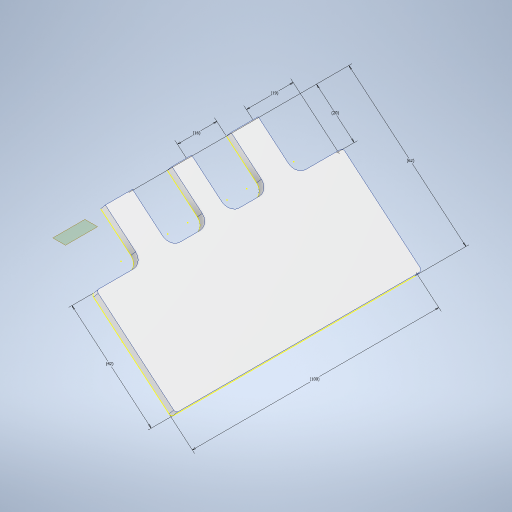
# Autodesk Inventor part: mirror
Saved by Autodesk Inventor 2023.5 (Build 275446000, 446)
## iProperties
Created: 2022-12-26
Part Number: mirror
Material: Aluminium 6061
Document SubType Name: Modeling
Designer: Kamil
Density: 2.7 g/cm^3
Appearance: Aluminium — płaski
Mass: 39.0399 g
Surface Area: 108.154 cm^2
Volume: 14.4592 cm^3
Author: Kamil
Autodesk Inventor part; units mm, degrees
ref_plane "YZ Plane" through (0, 0, 0) normal (1, 0, 0) x (0, 1, 0)
ref_plane "XZ Plane" through (0, 0, 0) normal (0, 1, 0) x (-1, 0, 0)
sketch "Sketch1" plane through (0, 0, 0) normal (0, 0, 1) x (1, 0, 0)
  line L0 (-44.6274, 16.55) -> (3.1619, -23.55) projected
  line L1 (44.6274, -23.55) -> (3.1619, -23.55) projected
  line L2 (44.6274, -23.55) -> (44.6274, -12.55) projected
  line L3 (44.6274, -12.55) -> (28.5274, -12.55) projected
  arc A0 (10.4274, 5.55) -> (28.5274, -12.55) centre (28.5274, 5.55) ccw projected
  line L4 (10.4274, 5.55) -> (10.4274, 16.55) projected
  line L5 (10.4274, 16.55) -> (-44.6274, 16.55) projected
  line L6 (-55.3726, 21.65) -> (-32.3912, 2.3664) projected
  line L7 (-32.3912, 2.3664) -> (-30.4629, 4.6645) projected
  line L8 (-30.4629, 4.6645) -> (-50.7054, 21.65) projected
  line L9 (-50.7054, 21.65) -> (-55.3726, 21.65) projected
  line L10 (-32.3912, 2.3664) -> (12.526, -35.3237)
  line L11 (3.1619, -23.55) -> (14.4544, -33.0256)
  line L12 (14.4544, -33.0256) -> (12.526, -35.3237)
  point P0 (0, 0)
  constraints: 6 end point, 1 perpendicular
ref_plane "Work Plane1" through (-44.6274, -23.55, -100) normal (0, 0, -1) x (0, 1, 0)
extrude "Extrusion1" add sketch "Sketch1" against normal up to surface (100 mm away) contours L0 L11 L12 L10 L7
sketch "Sketch2" plane through (14.4544, -33.0256, -100) normal (0, 0, -1) x (-0.7660444, 0.6427876, 0)
  line L0 (-13.6181, 16.6167) -> (-12.086, 15.3311)
  line L1 (-12.086, 15.3311) -> (12.4819, -5.2838)
  line L2 (0, 0) -> (58.6353, 0) projected
  line L3 (0, -3) -> (0, 0) projected
  line L4 (58.6353, -3) -> (0, -3) projected
  line L5 (58.6353, 0) -> (58.6353, -3) projected
  point P0 (32.3011, 16.0079)
  point P1 (9.7601, -3)
  point P2 (6.1849, 0)
  constraints: 4 end point, 3 other
extrude "Extrusion2" cut sketch "Sketch2" against normal through all contours L1 L4 L3 L2
ref_plane "Work Plane2" through (-55.2717, 8.4367, -43.1782) normal (0, -1, 0) x (1, 0, 0)
sketch "Sketch4" plane through (-32.3912, 2.3664, -100) normal (-0.6427876, -0.7660444, 0) x (0.7660444, -0.6427876, 0)
  line L0 (48.8752, 0) -> (48.8752, 100) projected
  line L1 (0, 100) -> (48.8752, 100) projected
  line L2 (0, 100) -> (0, 0) projected
  line L3 (0, 0) -> (48.8752, 0) projected
  line L4 (-5.8685, 94) -> (-21.784, 94)
  line L5 (43.894, 94) -> (0.9766, 94)
  line L6 (48.8752, 0) -> (48.8752, 100) projected
  line L7 (48.8752, 50) -> (0, 50)
  line L8 (0, 100) -> (0, 0) projected
  line L9 (26.3342, 100) -> (26.3342, 94)
  line L10 (26.3342, 97) -> (26.3342, 96.5)
  circle A0 centre (26.3342, 96.5) radius 1.5
  circle A1 centre (26.3342, 3.5) radius 1.5
  dimension "d6" = 0.5
  dimension "d7" = 3
  constraints: 10 end point, 3 midpoint, 2 centre point, 2 horizontal, 2 point on line, 1 coincident, 1 perpendicular, 1 symmetric about line, 5 other
  measures "d6" distance of L10.start L10.end
  measures "d7" diameter of A0
extrude "Extrusion3" cut sketch "Sketch4" against normal blind 10 contours L9 A0 | L9 A0 | A1
chamfer "Chamfer1" distance 1 angle 45 2 edges at (-13.3671, -13.5967, -3.5) (-13.3671, -13.5967, -96.5)
sketch "Szkic5" plane through (-32.3912, 2.3664, -100) normal (-0.7660444, 0.6427876, 0) x (0, 0, 1)
  line L0 (0, 3) -> (0, 0) projected
  line L1 (100, 0) -> (0, 0) projected
  line L2 (100, 3) -> (100, 0) projected
  line L3 (100, 3) -> (0, 3) projected
  point P0 (100, 19.0079)
extrude "Wyciągnięcie proste4" add sketch "Szkic5" along normal blind 10
sketch "Szkic6" plane through (5.0493, -29.05, -100) normal (-0.6427876, -0.7660444, 0) x (0.7660444, -0.6427876, 0)
  line L0 (-58.8752, 0) -> (-58.8752, 100) projected
  line L1 (-58.8752, 100) -> (0, 100) projected
  line L2 (0, 0) -> (-58.8752, 0) projected
  line L3 (-38.8752, 100) -> (-38.8752, 0)
  line L4 (-38.8752, 50) -> (-58.8752, 50)
  line L5 (-58.8752, 100) -> (-58.8752, 0) projected
  line L6 (-38.8752, 46) -> (-58.8752, 46)
  line L7 (-38.8752, 54) -> (-58.8752, 54)
  line L8 (-38.8752, 81) -> (-58.8752, 81)
  line L9 (-38.8752, 19) -> (-58.8752, 19)
  line L10 (-38.8752, 70) -> (-58.8752, 70)
  line L11 (-38.8752, 30) -> (-58.8752, 30)
  point P0 (-22.541, 100)
  point P1 (-58.8752, 19)
  point P2 (-58.8752, 30)
  point P3 (-58.8752, 46)
  point P4 (-58.8752, 54)
  point P5 (-58.8752, 81)
  dimension "d15" = 20
  dimension "d16" = 4
  dimension "d17" = 4
  dimension "d18" = 19
  dimension "d19" = 19
  dimension "d20" = 11
  dimension "d21" = 11
  constraints: 16 end point, 10 point on line, 5 perpendicular, 2 midpoint, 2 parallel
  measures "d15" distance between parallel lines of L0 L3
  measures "d16" distance between parallel lines of L4 L6
  measures "d17" distance between parallel lines of L4 L7
  measures "d18" distance between parallel lines of L8 L1
  measures "d19" distance between parallel lines of L2 L9
  measures "d20" distance between parallel lines of L9 L11
  measures "d21" distance between parallel lines of L8 L10
extrude "Wyciągnięcie proste5" cut sketch "Szkic6" against normal through all contours L0 L9 L3 L2 | L0 L6 L3 L11 | L0 L10 L3 L7 | L0 L1 L3 L8
fillet "Zaokrąglenie1" radius 4 6 edges at (-23.7666, -2.9124, -19) (-23.7666, -2.9124, -46) (-23.7666, -2.9124, -30) (-23.7666, -2.9124, -54) (-23.7666, -2.9124, -70) (-23.7666, -2.9124, -81)
sketch "Szkic7" plane through (5.0493, -29.05, -100) normal (-0.6427876, -0.7660444, 0) x (0.7660444, -0.6427876, 0)
  circle A0 centre (-22.541, 96.5) radius 2.5 projected
  circle A1 centre (-22.541, 3.5) radius 2.5 projected
  point P0 (-22.541, 100)
extrude "Wyciągnięcie proste6" add sketch "Szkic7" against normal up to surface (3 mm away)
sketch "Szkic8" plane through (5.0493, -29.05, -100) normal (-0.6427876, -0.7660444, 0) x (0.7660444, -0.6427876, 0)
  line L0 (-42.8752, 30) -> (-58.8752, 30) projected
  line L1 (-58.8752, 19) -> (-58.8752, 30) projected
  line L2 (-58.8752, 19) -> (-42.8752, 19) projected
  arc A0 (-38.8752, 15) -> (-42.8752, 19) centre (-42.8752, 15) ccw projected
  line L3 (-38.8752, 15) -> (-38.8752, 0) projected
  line L4 (0, 0) -> (-38.8752, 0) projected
  line L5 (0, 0) -> (0, 100) projected
  line L6 (-38.8752, 100) -> (0, 100) projected
  line L7 (-38.8752, 100) -> (-38.8752, 85) projected
  arc A1 (-42.8752, 81) -> (-38.8752, 85) centre (-42.8752, 85) ccw projected
  line L8 (-42.8752, 81) -> (-58.8752, 81) projected
  line L9 (-58.8752, 70) -> (-58.8752, 81) projected
  line L10 (-58.8752, 70) -> (-42.8752, 70) projected
  arc A2 (-38.8752, 66) -> (-42.8752, 70) centre (-42.8752, 66) ccw projected
  line L11 (-38.8752, 66) -> (-38.8752, 58) projected
  arc A3 (-42.8752, 54) -> (-38.8752, 58) centre (-42.8752, 58) ccw projected
  line L12 (-42.8752, 54) -> (-58.8752, 54) projected
  line L13 (-58.8752, 46) -> (-58.8752, 54) projected
  line L14 (-58.8752, 46) -> (-42.8752, 46) projected
  arc A4 (-38.8752, 42) -> (-42.8752, 46) centre (-42.8752, 42) ccw projected
  line L15 (-38.8752, 42) -> (-38.8752, 34) projected
  arc A5 (-42.8752, 30) -> (-38.8752, 34) centre (-42.8752, 34) ccw projected
  line L16 (0, 100) -> (3.5753, 100) projected
  line L17 (0, 0) -> (0, 100) projected
  line L18 (3.5753, 0) -> (0, 0) projected
  line L19 (3.5753, 100) -> (3.5753, 0) projected
  line L20 (3.5753, 100) -> (-38.8752, 100) projected
  line L21 (3.1248, 100) -> (3.1248, 0)
  line L22 (3.5753, 0) -> (-38.8752, 0) projected
  point P0 (-22.541, 100)
  point P1 (3.1248, 0)
  point P2 (3.1248, 100)
  point P3 (0, 100)
  point P4 (0, 0)
  dimension "d27" = 62
  constraints: 2 end point, 2 point on line, 1 perpendicular
  measures "d27" distance between parallel lines of L1 L21
extrude "Wyciągnięcie proste7" add sketch "Szkic8" along normal up to surface contours L5 L16 L21 L18 surface through (9.7165, -29.05, -100) normal (0, 1, 0)
extrude "Wyciągnięcie proste8" cut sketch "Szkic8" against normal through all contours L21 L16 L19 L18
fillet "Zaokrąglenie2" radius 1 4 edges at (-23.7666, -2.9124, 0) (8.4073, -29.9095, 0) (-23.7666, -2.9124, -100) (8.4073, -29.9095, -100)
sketch "Szkic9" plane through (-40.0517, 8.7942, -30) normal (-0.6427876, -0.7660444, 0) x (0.7660444, -0.6427876, 0)
  arc A0 (61, -70) -> (62, -69) centre (61, -69) ccw projected
  line L0 (62, -69) -> (62, 29) projected
  arc A1 (62, 29) -> (61, 30) centre (61, 29) ccw projected
  line L1 (21, 30) -> (61, 30) projected
  arc A2 (21, 30) -> (20, 29) centre (21, 29) ccw projected
  line L2 (20, 29) -> (20, 15) projected
  arc A3 (16, 11) -> (20, 15) centre (16, 15) ccw projected
  line L3 (16, 11) -> (0, 11) projected
  line L4 (0, 0) -> (0, 11) projected
  line L5 (0, 0) -> (16, 0) projected
  arc A4 (20, -4) -> (16, 0) centre (16, -4) ccw projected
  line L6 (20, -4) -> (20, -12) projected
  arc A5 (16, -16) -> (20, -12) centre (16, -12) ccw projected
  line L7 (16, -16) -> (0, -16) projected
  line L8 (0, -24) -> (0, -16) projected
  line L9 (0, -24) -> (16, -24) projected
  arc A6 (20, -28) -> (16, -24) centre (16, -28) ccw projected
  line L10 (20, -28) -> (20, -36) projected
  arc A7 (16, -40) -> (20, -36) centre (16, -36) ccw projected
  line L11 (16, -40) -> (0, -40) projected
  line L12 (0, -51) -> (0, -40) projected
  line L13 (0, -51) -> (16, -51) projected
  arc A8 (20, -55) -> (16, -51) centre (16, -55) ccw projected
  line L14 (20, -55) -> (20, -69) projected
  arc A9 (20, -69) -> (21, -70) centre (21, -69) ccw projected
  line L15 (21, -70) -> (61, -70) projected
  line L16 (0, 0) -> (0, 11) projected
  line L17 (62, -69) -> (62, 29) projected
  point P0 (36.3342, 30)
  dimension "d33" = 100
  dimension "d34" = 42
  dimension "d35" = 62
  dimension "d36" = 19
  dimension "d37" = 20
  dimension "d38" = 16
  measures "d33" distance between parallel lines of L15 L1
  measures "d34" distance between parallel lines of L2 L0
  measures "d35" distance between parallel lines of L4 L0
  measures "d36" distance between parallel lines of L15 L13
  measures "d37" distance between parallel lines of L12 L14
  measures "d38" distance between parallel lines of L11 L9
body "Solid1"
